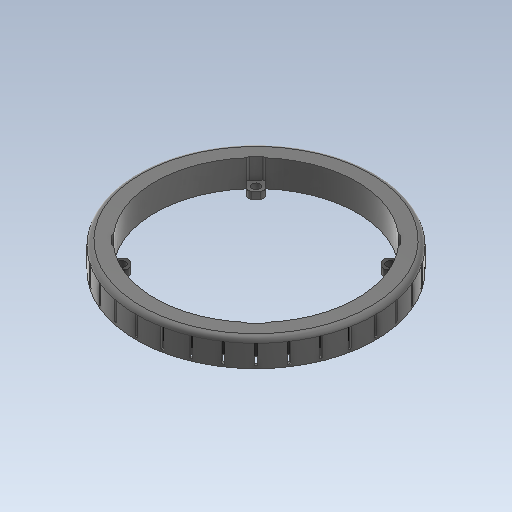
# Autodesk Inventor part: tsop_head
Saved by Autodesk Inventor 2020 (Build 240168000, 168)
## iProperties
Created: 2024-03-11
Part Number: tsop_head
Material: Типовые
Document SubType Name: Modeling
Designer: 4s
Density: 1 g/cm^3
Appearance: Гладкая — черная
Author: 4s
Autodesk Inventor part; units mm, degrees
ref_plane "YZ Plane" through (0, 0, 0) normal (1, 0, 0) x (0, 1, 0)
ref_plane "XZ Plane" through (0, 0, 0) normal (0, 1, 0) x (-1, 0, 0)
ref_plane "XY Plane" through (0, 0, 0) normal (0, 0, 1) x (1, 0, 0)
sketch "Эскиз1" plane through (0, 0, 0) normal (0, 1, 0) x (-1, 0, 0)
  circle A0 centre (0, 0) radius 44 construction
  line L0 (45.8, 2.65) -> (42.7, 2.65)
  line L1 (42.7, 2.65) -> (42.7, -2.65)
  line L2 (42.7, -2.65) -> (45.8, -2.65)
  line L3 (47.8, -0.65) -> (47.8, 0.65)
  line L4 (0, 0) -> (44, 0) construction
  line L5 (0, 0) -> (0, -44) construction
  circle A1 centre (0, 0) radius 49 construction
  circle A2 centre (0, 0) radius 42 construction
  circle A3 centre (0, 0) radius 39 construction
  arc A4 (47.8, 0.65) -> (45.8, 2.65) centre (45.8, 0.65) ccw
  arc A5 (45.8, -2.65) -> (47.8, -0.65) centre (45.8, -0.65) ccw
  line L6 (0, 0) -> (47.8, -0.4878) construction
  line L7 (0, 0) -> (47.8, 0.4878) construction
  line L8 (47.8, 0.4878) -> (48.9974, 0.5)
  line L9 (47.8, -0.4878) -> (48.9974, -0.5)
  line L10 (48.9974, 0.5) -> (49.2908, 0.1398)
  line L11 (49.2908, 0.1398) -> (48.9974, -0.5)
  arc A6 (48.9974, -0.5) -> (48.9974, 0.5) centre (0, 0) ccw
  point P0 (47.8, 2.65)
  point P1 (47.8, -2.65)
  point P2 (49, 0)
  dimension "d0" = 88
  dimension "d1" = 5.3
  dimension "d2" = 1.3
  dimension "d3" = 5.1
  dimension "d4" = 98
  dimension "d5" = 84
  dimension "d6" = 78
  dimension "d16" = 2
  dimension "d17" = 1
  constraints: 24 end point, 11 point on circle, 7 centre point, 6 point on line, 5 coincident, 4 tangent, 2 collinear, 2 horizontal, 2 parallel, 2 perpendicular, 1 equal radius, 1 symmetric about line, 1 other
  measures "d0" diameter of A0
  measures "d1" distance of point (47.8, -2.65) point (47.8, 2.65)
  measures "d2" distance from line of L4.end L1
  measures "d3" distance of L1.end point (47.8, -2.65)
  measures "d4" diameter of A1
  measures "d5" diameter of A2
  measures "d6" diameter of A3
  measures "d16" radius of A4
  measures "d17" distance of L8.end L9.end
sketch "Эскиз2" plane through (0, 0, 0) normal (0, 1, 0) x (-1, 0, 0)
  circle A0 centre (0, 0) radius 49
  circle A1 centre (0, 0) radius 42
  dimension "d7" = 98
  dimension "d8" = 84
  constraints: 2 centre point, 2 coincident
  measures "d7" diameter of A0
  measures "d8" diameter of A1
extrude "Выдавливание1" add sketch "Эскиз2" along normal blind 10
extrude "Выдавливание2" cut sketch "Эскиз1" along normal blind 10 contours A4 L3 A5 L2 L1 L0 | L10 L11 A6
pattern_circular "Круговой массив1" count 32 over 360 about axis through (0, 0, 0) along (0, 1, 0) of "Выдавливание2"
sketch "Эскиз3" plane through (0, 10, 0) normal (0, 1, 0) x (1, 0, 0)
  line L0 (-47.8, -0.65) -> (-47.8, 0.65) construction
  arc A0 (-45.8, 2.65) -> (-47.8, 0.65) centre (-45.8, 0.65) ccw construction
  line L1 (-45.8, 2.65) -> (-42.7, 2.65) construction
  line L2 (-42.7, 2.65) -> (-42.7, -2.65) construction
  line L3 (-42.7, -2.65) -> (-45.8, -2.65) construction
  arc A1 (-47.8, -0.65) -> (-45.8, -2.65) centre (-45.8, -0.65) ccw construction
  line L4 (-46.7547, -9.9628) -> (-47.0083, -8.6878) construction
  arc A2 (-45.437, -6.3361) -> (-47.0083, -8.6878) centre (-45.0468, -8.2976) ccw construction
  line L5 (-45.437, -6.3361) -> (-42.3965, -5.7313) construction
  line L6 (-42.3965, -5.7313) -> (-41.3625, -10.9294) construction
  line L7 (-41.3625, -10.9294) -> (-44.403, -11.5342) construction
  arc A3 (-46.7547, -9.9628) -> (-44.403, -11.5342) centre (-44.7932, -9.5726) ccw construction
  line L8 (-43.9127, -18.8928) -> (-44.4102, -17.6917) construction
  arc A4 (-43.3278, -15.0786) -> (-44.4102, -17.6917) centre (-42.5624, -16.9264) ccw construction
  line L9 (-43.3278, -15.0786) -> (-40.4638, -13.8923) construction
  line L10 (-40.4638, -13.8923) -> (-38.4355, -18.7889) construction
  line L11 (-38.4355, -18.7889) -> (-41.2996, -19.9752) construction
  arc A5 (-43.9127, -18.8928) -> (-41.2996, -19.9752) centre (-42.0649, -18.1274) ccw construction
  line L12 (-39.3831, -27.0967) -> (-40.1054, -26.0158) construction
  arc A6 (-39.5536, -23.2417) -> (-40.1054, -26.0158) centre (-38.4424, -24.9047) ccw construction
  line L13 (-39.5536, -23.2417) -> (-36.976, -21.5195) construction
  line L14 (-36.976, -21.5195) -> (-34.0315, -25.9262) construction
  line L15 (-34.0315, -25.9262) -> (-36.609, -27.6485) construction
  arc A7 (-39.3831, -27.0967) -> (-36.609, -27.6485) centre (-37.7202, -25.9856) ccw construction
  line L16 (-33.3401, -34.2593) -> (-34.2593, -33.3401) construction
  arc A8 (-34.2593, -30.5117) -> (-34.2593, -33.3401) centre (-32.8451, -31.9259) ccw construction
  line L17 (-34.2593, -30.5117) -> (-32.0673, -28.3196) construction
  line L18 (-32.0673, -28.3196) -> (-28.3196, -32.0673) construction
  line L19 (-28.3196, -32.0673) -> (-30.5117, -34.2593) construction
  arc A9 (-33.3401, -34.2593) -> (-30.5117, -34.2593) centre (-31.9259, -32.8451) ccw construction
  line L20 (-26.0158, -40.1054) -> (-27.0967, -39.3831) construction
  arc A10 (-27.6485, -36.609) -> (-27.0967, -39.3831) centre (-25.9856, -37.7202) ccw construction
  line L21 (-27.6485, -36.609) -> (-25.9262, -34.0315) construction
  line L22 (-25.9262, -34.0315) -> (-21.5195, -36.976) construction
  line L23 (-21.5195, -36.976) -> (-23.2417, -39.5536) construction
  arc A11 (-26.0158, -40.1054) -> (-23.2417, -39.5536) centre (-24.9047, -38.4424) ccw construction
  line L24 (-17.6917, -44.4102) -> (-18.8928, -43.9127) construction
  arc A12 (-19.9752, -41.2996) -> (-18.8928, -43.9127) centre (-18.1274, -42.0649) ccw construction
  line L25 (-19.9752, -41.2996) -> (-18.7889, -38.4355) construction
  line L26 (-18.7889, -38.4355) -> (-13.8923, -40.4638) construction
  line L27 (-13.8923, -40.4638) -> (-15.0786, -43.3278) construction
  arc A13 (-17.6917, -44.4102) -> (-15.0786, -43.3278) centre (-16.9264, -42.5624) ccw construction
  line L28 (-8.6878, -47.0083) -> (-9.9628, -46.7547) construction
  arc A14 (-11.5342, -44.403) -> (-9.9628, -46.7547) centre (-9.5726, -44.7932) ccw construction
  line L29 (-11.5342, -44.403) -> (-10.9294, -41.3625) construction
  line L30 (-10.9294, -41.3625) -> (-5.7313, -42.3965) construction
  line L31 (-5.7313, -42.3965) -> (-6.3361, -45.437) construction
  arc A15 (-8.6878, -47.0083) -> (-6.3361, -45.437) centre (-8.2976, -45.0468) ccw construction
  line L32 (0.65, -47.8) -> (-0.65, -47.8) construction
  arc A16 (-2.65, -45.8) -> (-0.65, -47.8) centre (-0.65, -45.8) ccw construction
  line L33 (-2.65, -45.8) -> (-2.65, -42.7) construction
  line L34 (-2.65, -42.7) -> (2.65, -42.7) construction
  line L35 (2.65, -42.7) -> (2.65, -45.8) construction
  arc A17 (0.65, -47.8) -> (2.65, -45.8) centre (0.65, -45.8) ccw construction
  line L36 (9.9628, -46.7547) -> (8.6878, -47.0083) construction
  arc A18 (6.3361, -45.437) -> (8.6878, -47.0083) centre (8.2976, -45.0468) ccw construction
  line L37 (6.3361, -45.437) -> (5.7313, -42.3965) construction
  line L38 (5.7313, -42.3965) -> (10.9294, -41.3625) construction
  line L39 (10.9294, -41.3625) -> (11.5342, -44.403) construction
  arc A19 (9.9628, -46.7547) -> (11.5342, -44.403) centre (9.5726, -44.7932) ccw construction
  line L40 (18.8928, -43.9127) -> (17.6917, -44.4102) construction
  arc A20 (15.0786, -43.3278) -> (17.6917, -44.4102) centre (16.9264, -42.5624) ccw construction
  line L41 (15.0786, -43.3278) -> (13.8923, -40.4638) construction
  line L42 (13.8923, -40.4638) -> (18.7889, -38.4355) construction
  line L43 (18.7889, -38.4355) -> (19.9752, -41.2996) construction
  arc A21 (18.8928, -43.9127) -> (19.9752, -41.2996) centre (18.1274, -42.0649) ccw construction
  line L44 (27.0967, -39.3831) -> (26.0158, -40.1054) construction
  arc A22 (23.2417, -39.5536) -> (26.0158, -40.1054) centre (24.9047, -38.4424) ccw construction
  line L45 (23.2417, -39.5536) -> (21.5195, -36.976) construction
  line L46 (21.5195, -36.976) -> (25.9262, -34.0315) construction
  line L47 (25.9262, -34.0315) -> (27.6485, -36.609) construction
  arc A23 (27.0967, -39.3831) -> (27.6485, -36.609) centre (25.9856, -37.7202) ccw construction
  line L48 (34.2593, -33.3401) -> (33.3401, -34.2593) construction
  arc A24 (30.5117, -34.2593) -> (33.3401, -34.2593) centre (31.9259, -32.8451) ccw construction
  line L49 (30.5117, -34.2593) -> (28.3196, -32.0673) construction
  line L50 (28.3196, -32.0673) -> (32.0673, -28.3196) construction
  line L51 (32.0673, -28.3196) -> (34.2593, -30.5117) construction
  arc A25 (34.2593, -33.3401) -> (34.2593, -30.5117) centre (32.8451, -31.9259) ccw construction
  line L52 (40.1054, -26.0158) -> (39.3831, -27.0967) construction
  arc A26 (36.609, -27.6485) -> (39.3831, -27.0967) centre (37.7202, -25.9856) ccw construction
  line L53 (36.609, -27.6485) -> (34.0315, -25.9262) construction
  line L54 (34.0315, -25.9262) -> (36.976, -21.5195) construction
  line L55 (36.976, -21.5195) -> (39.5536, -23.2417) construction
  arc A27 (40.1054, -26.0158) -> (39.5536, -23.2417) centre (38.4424, -24.9047) ccw construction
  line L56 (44.4102, -17.6917) -> (43.9127, -18.8928) construction
  arc A28 (41.2996, -19.9752) -> (43.9127, -18.8928) centre (42.0649, -18.1274) ccw construction
  line L57 (41.2996, -19.9752) -> (38.4355, -18.7889) construction
  line L58 (38.4355, -18.7889) -> (40.4638, -13.8923) construction
  line L59 (40.4638, -13.8923) -> (43.3278, -15.0786) construction
  arc A29 (44.4102, -17.6917) -> (43.3278, -15.0786) centre (42.5624, -16.9264) ccw construction
  line L60 (47.0083, -8.6878) -> (46.7547, -9.9628) construction
  arc A30 (44.403, -11.5342) -> (46.7547, -9.9628) centre (44.7932, -9.5726) ccw construction
  line L61 (44.403, -11.5342) -> (41.3625, -10.9294) construction
  line L62 (41.3625, -10.9294) -> (42.3965, -5.7313) construction
  line L63 (42.3965, -5.7313) -> (45.437, -6.3361) construction
  arc A31 (47.0083, -8.6878) -> (45.437, -6.3361) centre (45.0468, -8.2976) ccw construction
  line L64 (47.8, 0.65) -> (47.8, -0.65) construction
  arc A32 (45.8, -2.65) -> (47.8, -0.65) centre (45.8, -0.65) ccw construction
  line L65 (45.8, -2.65) -> (42.7, -2.65) construction
  line L66 (42.7, -2.65) -> (42.7, 2.65) construction
  line L67 (42.7, 2.65) -> (45.8, 2.65) construction
  arc A33 (47.8, 0.65) -> (45.8, 2.65) centre (45.8, 0.65) ccw construction
  line L68 (46.7547, 9.9628) -> (47.0083, 8.6878) construction
  arc A34 (45.437, 6.3361) -> (47.0083, 8.6878) centre (45.0468, 8.2976) ccw construction
  line L69 (45.437, 6.3361) -> (42.3965, 5.7313) construction
  line L70 (42.3965, 5.7313) -> (41.3625, 10.9294) construction
  line L71 (41.3625, 10.9294) -> (44.403, 11.5342) construction
  arc A35 (46.7547, 9.9628) -> (44.403, 11.5342) centre (44.7932, 9.5726) ccw construction
  line L72 (43.9127, 18.8928) -> (44.4102, 17.6917) construction
  arc A36 (43.3278, 15.0786) -> (44.4102, 17.6917) centre (42.5624, 16.9264) ccw construction
  line L73 (43.3278, 15.0786) -> (40.4638, 13.8923) construction
  line L74 (40.4638, 13.8923) -> (38.4355, 18.7889) construction
  line L75 (38.4355, 18.7889) -> (41.2996, 19.9752) construction
  arc A37 (43.9127, 18.8928) -> (41.2996, 19.9752) centre (42.0649, 18.1274) ccw construction
  line L76 (39.3831, 27.0967) -> (40.1054, 26.0158) construction
  arc A38 (39.5536, 23.2417) -> (40.1054, 26.0158) centre (38.4424, 24.9047) ccw construction
  line L77 (39.5536, 23.2417) -> (36.976, 21.5195) construction
  line L78 (36.976, 21.5195) -> (34.0315, 25.9262) construction
  line L79 (34.0315, 25.9262) -> (36.609, 27.6485) construction
  arc A39 (39.3831, 27.0967) -> (36.609, 27.6485) centre (37.7202, 25.9856) ccw construction
  line L80 (33.3401, 34.2593) -> (34.2593, 33.3401) construction
  arc A40 (34.2593, 30.5117) -> (34.2593, 33.3401) centre (32.8451, 31.9259) ccw construction
  line L81 (34.2593, 30.5117) -> (32.0673, 28.3196) construction
  line L82 (32.0673, 28.3196) -> (28.3196, 32.0673) construction
  line L83 (28.3196, 32.0673) -> (30.5117, 34.2593) construction
  arc A41 (33.3401, 34.2593) -> (30.5117, 34.2593) centre (31.9259, 32.8451) ccw construction
  line L84 (26.0158, 40.1054) -> (27.0967, 39.3831) construction
  arc A42 (27.6485, 36.609) -> (27.0967, 39.3831) centre (25.9856, 37.7202) ccw construction
  line L85 (27.6485, 36.609) -> (25.9262, 34.0315) construction
  line L86 (25.9262, 34.0315) -> (21.5195, 36.976) construction
  line L87 (21.5195, 36.976) -> (23.2417, 39.5536) construction
  arc A43 (26.0158, 40.1054) -> (23.2417, 39.5536) centre (24.9047, 38.4424) ccw construction
  line L88 (17.6917, 44.4102) -> (18.8928, 43.9127) construction
  arc A44 (19.9752, 41.2996) -> (18.8928, 43.9127) centre (18.1274, 42.0649) ccw construction
  line L89 (19.9752, 41.2996) -> (18.7889, 38.4355) construction
  line L90 (18.7889, 38.4355) -> (13.8923, 40.4638) construction
  line L91 (13.8923, 40.4638) -> (15.0786, 43.3278) construction
  arc A45 (17.6917, 44.4102) -> (15.0786, 43.3278) centre (16.9264, 42.5624) ccw construction
  line L92 (8.6878, 47.0083) -> (9.9628, 46.7547) construction
  arc A46 (11.5342, 44.403) -> (9.9628, 46.7547) centre (9.5726, 44.7932) ccw construction
  line L93 (11.5342, 44.403) -> (10.9294, 41.3625) construction
  line L94 (10.9294, 41.3625) -> (5.7313, 42.3965) construction
  line L95 (5.7313, 42.3965) -> (6.3361, 45.437) construction
  arc A47 (8.6878, 47.0083) -> (6.3361, 45.437) centre (8.2976, 45.0468) ccw construction
  line L96 (-0.65, 47.8) -> (0.65, 47.8) construction
  arc A48 (2.65, 45.8) -> (0.65, 47.8) centre (0.65, 45.8) ccw construction
  line L97 (2.65, 45.8) -> (2.65, 42.7) construction
  line L98 (2.65, 42.7) -> (-2.65, 42.7) construction
  line L99 (-2.65, 42.7) -> (-2.65, 45.8) construction
  arc A49 (-0.65, 47.8) -> (-2.65, 45.8) centre (-0.65, 45.8) ccw construction
  line L100 (-9.9628, 46.7547) -> (-8.6878, 47.0083) construction
  arc A50 (-6.3361, 45.437) -> (-8.6878, 47.0083) centre (-8.2976, 45.0468) ccw construction
  line L101 (-6.3361, 45.437) -> (-5.7313, 42.3965) construction
  line L102 (-5.7313, 42.3965) -> (-10.9294, 41.3625) construction
  line L103 (-10.9294, 41.3625) -> (-11.5342, 44.403) construction
  arc A51 (-9.9628, 46.7547) -> (-11.5342, 44.403) centre (-9.5726, 44.7932) ccw construction
  line L104 (-18.8928, 43.9127) -> (-17.6917, 44.4102) construction
  arc A52 (-15.0786, 43.3278) -> (-17.6917, 44.4102) centre (-16.9264, 42.5624) ccw construction
  line L105 (-15.0786, 43.3278) -> (-13.8923, 40.4638) construction
  line L106 (-13.8923, 40.4638) -> (-18.7889, 38.4355) construction
  line L107 (-18.7889, 38.4355) -> (-19.9752, 41.2996) construction
  arc A53 (-18.8928, 43.9127) -> (-19.9752, 41.2996) centre (-18.1274, 42.0649) ccw construction
  line L108 (-27.0967, 39.3831) -> (-26.0158, 40.1054) construction
  arc A54 (-23.2417, 39.5536) -> (-26.0158, 40.1054) centre (-24.9047, 38.4424) ccw construction
  line L109 (-23.2417, 39.5536) -> (-21.5195, 36.976) construction
  line L110 (-21.5195, 36.976) -> (-25.9262, 34.0315) construction
  line L111 (-25.9262, 34.0315) -> (-27.6485, 36.609) construction
  arc A55 (-27.0967, 39.3831) -> (-27.6485, 36.609) centre (-25.9856, 37.7202) ccw construction
  line L112 (-34.2593, 33.3401) -> (-33.3401, 34.2593) construction
  arc A56 (-30.5117, 34.2593) -> (-33.3401, 34.2593) centre (-31.9259, 32.8451) ccw construction
  line L113 (-30.5117, 34.2593) -> (-28.3196, 32.0673) construction
  line L114 (-28.3196, 32.0673) -> (-32.0673, 28.3196) construction
  line L115 (-32.0673, 28.3196) -> (-34.2593, 30.5117) construction
  arc A57 (-34.2593, 33.3401) -> (-34.2593, 30.5117) centre (-32.8451, 31.9259) ccw construction
  line L116 (-40.1054, 26.0158) -> (-39.3831, 27.0967) construction
  arc A58 (-36.609, 27.6485) -> (-39.3831, 27.0967) centre (-37.7202, 25.9856) ccw construction
  line L117 (-36.609, 27.6485) -> (-34.0315, 25.9262) construction
  line L118 (-34.0315, 25.9262) -> (-36.976, 21.5195) construction
  line L119 (-36.976, 21.5195) -> (-39.5536, 23.2417) construction
  arc A59 (-40.1054, 26.0158) -> (-39.5536, 23.2417) centre (-38.4424, 24.9047) ccw construction
  line L120 (-44.4102, 17.6917) -> (-43.9127, 18.8928) construction
  arc A60 (-41.2996, 19.9752) -> (-43.9127, 18.8928) centre (-42.0649, 18.1274) ccw construction
  line L121 (-41.2996, 19.9752) -> (-38.4355, 18.7889) construction
  line L122 (-38.4355, 18.7889) -> (-40.4638, 13.8923) construction
  line L123 (-40.4638, 13.8923) -> (-43.3278, 15.0786) construction
  arc A61 (-44.4102, 17.6917) -> (-43.3278, 15.0786) centre (-42.5624, 16.9264) ccw construction
  line L124 (-47.0083, 8.6878) -> (-46.7547, 9.9628) construction
  arc A62 (-44.403, 11.5342) -> (-46.7547, 9.9628) centre (-44.7932, 9.5726) ccw construction
  line L125 (-44.403, 11.5342) -> (-41.3625, 10.9294) construction
  line L126 (-41.3625, 10.9294) -> (-42.3965, 5.7313) construction
  line L127 (-42.3965, 5.7313) -> (-45.437, 6.3361) construction
  arc A63 (-47.0083, 8.6878) -> (-45.437, 6.3361) centre (-45.0468, 8.2976) ccw construction
  circle A64 centre (0, 0) radius 42 projected
  circle A65 centre (0, 0) radius 49
  constraints: 1 centre point, 1 coincident
extrude "Выдавливание3" add sketch "Эскиз3" along normal blind 1
fillet "Сопряжение1" radius 2 1 edges at (-49, 11, 0)
extrude "Выдавливание4" cut sketch "Эскиз1" along normal blind 9 contours L8 A6 L9 L3
pattern_circular "Круговой массив2" count 32 over 360 about axis through (0, 0, 0) along (0, 1, 0) of "Выдавливание4"
fillet "Сопряжение2" radius 0.5 1 edges at (-46.8815, 9, -9.3253)
sketch "Эскиз4" plane through (0, 0, 0) normal (0, -1, 0) x (1, 0, 0)
  circle A0 centre (0, 0) radius 39 construction
  line L0 (0, 0) -> (-27.5772, -27.5772) construction
  line L1 (0, 0) -> (39, 0) construction
  circle A1 centre (-27.5772, -27.5772) radius 1.7
  line L2 (0, 0) -> (0, -39) construction
  circle A2 centre (27.5772, -27.5772) radius 1.7
  circle A3 centre (-27.5772, 27.5772) radius 1.7
  circle A4 centre (27.5772, 27.5772) radius 1.7
  line L3 (-31.5793, -27.6902) -> (-28.8146, -24.9255)
  line L4 (-27.6902, -31.5793) -> (-24.9255, -28.8146)
  circle A5 centre (0, 0) radius 42 construction
  circle A6 centre (0, 0) radius 47 construction
  circle A7 centre (0, 0) radius 42 construction
  line L5 (-26.6933, -24.9255) -> (-24.9255, -26.6933)
  arc A8 (-24.9255, -28.8146) -> (-24.9255, -26.6933) centre (-25.9862, -27.7539) ccw
  arc A9 (-26.6933, -24.9255) -> (-28.8146, -24.9255) centre (-27.7539, -25.9862) ccw
  arc A10 (-31.5793, -27.6902) -> (-27.6902, -31.5793) centre (0, 0) ccw
  point P0 (-39, 0)
  point P1 (0, 39)
  point P2 (-27.7539, -23.8649)
  point P3 (-23.8649, -27.7539)
  dimension "d27" = 78
  dimension "d28" = 135
  dimension "d29" = 3.4
  dimension "d30" = 5.5
  dimension "d31" = 2.5
  dimension "d32" = 1.5
  dimension "d33" = 42
  constraints: 12 end point, 11 point on circle, 8 centre point, 5 symmetric about line, 4 point on line, 4 tangent, 2 coincident, 1 equal length, 1 equal radius, 1 horizontal, 1 parallel, 1 vertical, 5 other
  measures "d27" diameter of A0
  measures "d28" angle of L0 L1
  measures "d29" diameter of A1
  measures "d30" distance between parallel lines of L3 L4
  measures "d31" distance from line of L0.end L5
  measures "d32" radius of A8
  measures "d33" radius of A10
extrude "Выдавливание5" add sketch "Эскиз4" along normal blind 0.3 and the other way blind 2.5 contours L3 A9 L5 A8 L4 A10
pattern_circular "Круговой массив3" count 4 over 360 about axis through (0, 0, 0) along (0, 1, 0) of "Выдавливание5"
sketch "Эскиз5" plane through (0, 0, 0) normal (0, -1, 0) x (1, 0, 0)
  circle A0 centre (0, 0) radius 47 construction
  line L0 (-46.7864, -9.8037) -> (-47.9584, -10.0493) construction
  arc A1 (-47.9584, -10.0493) -> (-45.4591, -18.2886) centre (0, 0) ccw construction
  line L1 (-45.4591, -18.2886) -> (-44.3481, -17.8416) construction
  line L2 (-44.3481, -17.8416) -> (-44.4102, -17.6917) construction
  arc A2 (-43.3278, -15.0786) -> (-44.4102, -17.6917) centre (-42.5624, -16.9264) ccw construction
  line L3 (-43.3278, -15.0786) -> (-40.4638, -13.8923) construction
  line L4 (-40.4638, -13.8923) -> (-38.4355, -18.7889) construction
  line L5 (-38.4355, -18.7889) -> (-41.2996, -19.9752) construction
  arc A3 (-43.9127, -18.8928) -> (-41.2996, -19.9752) centre (-42.0649, -18.1274) ccw construction
  line L6 (-43.9127, -18.8928) -> (-43.9748, -18.7429) construction
  line L7 (-43.9748, -18.7429) -> (-45.0764, -19.2125) construction
  arc A4 (-45.0764, -19.2125) -> (-41.0177, -26.8058) centre (0, 0) ccw construction
  line L8 (-41.0177, -26.8058) -> (-40.0152, -26.1507) construction
  line L9 (-40.0152, -26.1507) -> (-40.1054, -26.0158) construction
  arc A5 (-39.5536, -23.2417) -> (-40.1054, -26.0158) centre (-38.4424, -24.9047) ccw construction
  line L10 (-39.5536, -23.2417) -> (-36.976, -21.5195) construction
  line L11 (-36.976, -21.5195) -> (-34.0315, -25.9262) construction
  line L12 (-34.0315, -25.9262) -> (-36.609, -27.6485) construction
  arc A6 (-39.3831, -27.0967) -> (-36.609, -27.6485) centre (-37.7202, -25.9856) ccw construction
  line L13 (-39.3831, -27.0967) -> (-39.4733, -26.9618) construction
  line L14 (-39.4733, -26.9618) -> (-40.4621, -27.6373) construction
  arc A7 (-40.4621, -27.6373) -> (-35, -34.2929) centre (0, 0) ccw construction
  line L15 (-35, -34.2929) -> (-34.1446, -33.4548) construction
  line L16 (-34.1446, -33.4548) -> (-34.2593, -33.3401) construction
  arc A8 (-34.2593, -30.5117) -> (-34.2593, -33.3401) centre (-32.8451, -31.9259) ccw construction
  line L17 (-34.2593, -30.5117) -> (-32.0673, -28.3196) construction
  line L18 (-32.0673, -28.3196) -> (-28.3196, -32.0673) construction
  line L19 (-28.3196, -32.0673) -> (-30.5117, -34.2593) construction
  arc A9 (-33.3401, -34.2593) -> (-30.5117, -34.2593) centre (-31.9259, -32.8451) ccw construction
  line L20 (-33.3401, -34.2593) -> (-33.4548, -34.1446) construction
  line L21 (-33.4548, -34.1446) -> (-34.2929, -35) construction
  arc A10 (-34.2929, -35) -> (-27.6373, -40.4621) centre (0, 0) ccw construction
  line L22 (-27.6373, -40.4621) -> (-26.9618, -39.4733) construction
  line L23 (-26.9618, -39.4733) -> (-27.0967, -39.3831) construction
  arc A11 (-27.6485, -36.609) -> (-27.0967, -39.3831) centre (-25.9856, -37.7202) ccw construction
  line L24 (-27.6485, -36.609) -> (-25.9262, -34.0315) construction
  line L25 (-25.9262, -34.0315) -> (-21.5195, -36.976) construction
  line L26 (-21.5195, -36.976) -> (-23.2417, -39.5536) construction
  arc A12 (-26.0158, -40.1054) -> (-23.2417, -39.5536) centre (-24.9047, -38.4424) ccw construction
  line L27 (-26.0158, -40.1054) -> (-26.1507, -40.0152) construction
  line L28 (-26.1507, -40.0152) -> (-26.8058, -41.0177) construction
  arc A13 (-26.8058, -41.0177) -> (-19.2125, -45.0764) centre (0, 0) ccw construction
  line L29 (-19.2125, -45.0764) -> (-18.7429, -43.9748) construction
  line L30 (-18.7429, -43.9748) -> (-18.8928, -43.9127) construction
  arc A14 (-19.9752, -41.2996) -> (-18.8928, -43.9127) centre (-18.1274, -42.0649) ccw construction
  line L31 (-19.9752, -41.2996) -> (-18.7889, -38.4355) construction
  line L32 (-18.7889, -38.4355) -> (-13.8923, -40.4638) construction
  line L33 (-13.8923, -40.4638) -> (-15.0786, -43.3278) construction
  arc A15 (-17.6917, -44.4102) -> (-15.0786, -43.3278) centre (-16.9264, -42.5624) ccw construction
  line L34 (-17.6917, -44.4102) -> (-17.8416, -44.3481) construction
  line L35 (-17.8416, -44.3481) -> (-18.2886, -45.4591) construction
  arc A16 (-18.2886, -45.4591) -> (-10.0493, -47.9584) centre (0, 0) ccw construction
  line L36 (-10.0493, -47.9584) -> (-9.8037, -46.7864) construction
  line L37 (-9.8037, -46.7864) -> (-9.9628, -46.7547) construction
  arc A17 (-11.5342, -44.403) -> (-9.9628, -46.7547) centre (-9.5726, -44.7932) ccw construction
  line L38 (-11.5342, -44.403) -> (-10.9294, -41.3625) construction
  line L39 (-10.9294, -41.3625) -> (-5.7313, -42.3965) construction
  line L40 (-5.7313, -42.3965) -> (-6.3361, -45.437) construction
  arc A18 (-8.6878, -47.0083) -> (-6.3361, -45.437) centre (-8.2976, -45.0468) ccw construction
  line L41 (-8.6878, -47.0083) -> (-8.8469, -46.9767) construction
  line L42 (-8.8469, -46.9767) -> (-9.0685, -48.1535) construction
  arc A19 (-9.0685, -48.1535) -> (-0.5, -48.9974) centre (0, 0) ccw construction
  line L43 (-0.5, -48.9974) -> (-0.4878, -47.8) construction
  line L44 (-0.4878, -47.8) -> (-0.65, -47.8) construction
  arc A20 (-2.65, -45.8) -> (-0.65, -47.8) centre (-0.65, -45.8) ccw construction
  line L45 (-2.65, -45.8) -> (-2.65, -42.7) construction
  line L46 (-2.65, -42.7) -> (2.65, -42.7) construction
  line L47 (2.65, -42.7) -> (2.65, -45.8) construction
  arc A21 (0.65, -47.8) -> (2.65, -45.8) centre (0.65, -45.8) ccw construction
  line L48 (0.65, -47.8) -> (0.4878, -47.8) construction
  line L49 (0.4878, -47.8) -> (0.5, -48.9974) construction
  arc A22 (0.5, -48.9974) -> (9.0685, -48.1535) centre (0, 0) ccw construction
  line L50 (9.0685, -48.1535) -> (8.8469, -46.9767) construction
  line L51 (8.8469, -46.9767) -> (8.6878, -47.0083) construction
  arc A23 (6.3361, -45.437) -> (8.6878, -47.0083) centre (8.2976, -45.0468) ccw construction
  line L52 (6.3361, -45.437) -> (5.7313, -42.3965) construction
  line L53 (5.7313, -42.3965) -> (10.9294, -41.3625) construction
  line L54 (10.9294, -41.3625) -> (11.5342, -44.403) construction
  arc A24 (9.9628, -46.7547) -> (11.5342, -44.403) centre (9.5726, -44.7932) ccw construction
  line L55 (9.9628, -46.7547) -> (9.8037, -46.7864) construction
  line L56 (9.8037, -46.7864) -> (10.0493, -47.9584) construction
  arc A25 (10.0493, -47.9584) -> (18.2886, -45.4591) centre (0, 0) ccw construction
  line L57 (18.2886, -45.4591) -> (17.8416, -44.3481) construction
  line L58 (17.8416, -44.3481) -> (17.6917, -44.4102) construction
  arc A26 (15.0786, -43.3278) -> (17.6917, -44.4102) centre (16.9264, -42.5624) ccw construction
  line L59 (15.0786, -43.3278) -> (13.8923, -40.4638) construction
  line L60 (13.8923, -40.4638) -> (18.7889, -38.4355) construction
  line L61 (18.7889, -38.4355) -> (19.9752, -41.2996) construction
  arc A27 (18.8928, -43.9127) -> (19.9752, -41.2996) centre (18.1274, -42.0649) ccw construction
  line L62 (18.8928, -43.9127) -> (18.7429, -43.9748) construction
  line L63 (18.7429, -43.9748) -> (19.2125, -45.0764) construction
  arc A28 (19.2125, -45.0764) -> (26.8058, -41.0177) centre (0, 0) ccw construction
  line L64 (26.8058, -41.0177) -> (26.1507, -40.0152) construction
  line L65 (26.1507, -40.0152) -> (26.0158, -40.1054) construction
  arc A29 (23.2417, -39.5536) -> (26.0158, -40.1054) centre (24.9047, -38.4424) ccw construction
  line L66 (23.2417, -39.5536) -> (21.5195, -36.976) construction
  line L67 (21.5195, -36.976) -> (25.9262, -34.0315) construction
  line L68 (25.9262, -34.0315) -> (27.6485, -36.609) construction
  arc A30 (27.0967, -39.3831) -> (27.6485, -36.609) centre (25.9856, -37.7202) ccw construction
  line L69 (27.0967, -39.3831) -> (26.9618, -39.4733) construction
  line L70 (26.9618, -39.4733) -> (27.6373, -40.4621) construction
  arc A31 (27.6373, -40.4621) -> (34.2929, -35) centre (0, 0) ccw construction
  line L71 (34.2929, -35) -> (33.4548, -34.1446) construction
  line L72 (33.4548, -34.1446) -> (33.3401, -34.2593) construction
  arc A32 (30.5117, -34.2593) -> (33.3401, -34.2593) centre (31.9259, -32.8451) ccw construction
  line L73 (30.5117, -34.2593) -> (28.3196, -32.0673) construction
  line L74 (28.3196, -32.0673) -> (32.0673, -28.3196) construction
  line L75 (32.0673, -28.3196) -> (34.2593, -30.5117) construction
  arc A33 (34.2593, -33.3401) -> (34.2593, -30.5117) centre (32.8451, -31.9259) ccw construction
  line L76 (34.2593, -33.3401) -> (34.1446, -33.4548) construction
  line L77 (34.1446, -33.4548) -> (35, -34.2929) construction
  arc A34 (35, -34.2929) -> (40.4621, -27.6373) centre (0, 0) ccw construction
  line L78 (40.4621, -27.6373) -> (39.4733, -26.9618) construction
  line L79 (39.4733, -26.9618) -> (39.3831, -27.0967) construction
  arc A35 (36.609, -27.6485) -> (39.3831, -27.0967) centre (37.7202, -25.9856) ccw construction
  line L80 (36.609, -27.6485) -> (34.0315, -25.9262) construction
  line L81 (34.0315, -25.9262) -> (36.976, -21.5195) construction
  line L82 (36.976, -21.5195) -> (39.5536, -23.2417) construction
  arc A36 (40.1054, -26.0158) -> (39.5536, -23.2417) centre (38.4424, -24.9047) ccw construction
  line L83 (40.1054, -26.0158) -> (40.0152, -26.1507) construction
  line L84 (40.0152, -26.1507) -> (41.0177, -26.8058) construction
  arc A37 (41.0177, -26.8058) -> (45.0764, -19.2125) centre (0, 0) ccw construction
  line L85 (45.0764, -19.2125) -> (43.9748, -18.7429) construction
  line L86 (43.9748, -18.7429) -> (43.9127, -18.8928) construction
  arc A38 (41.2996, -19.9752) -> (43.9127, -18.8928) centre (42.0649, -18.1274) ccw construction
  line L87 (41.2996, -19.9752) -> (38.4355, -18.7889) construction
  line L88 (38.4355, -18.7889) -> (40.4638, -13.8923) construction
  line L89 (40.4638, -13.8923) -> (43.3278, -15.0786) construction
  arc A39 (44.4102, -17.6917) -> (43.3278, -15.0786) centre (42.5624, -16.9264) ccw construction
  line L90 (44.4102, -17.6917) -> (44.3481, -17.8416) construction
  line L91 (44.3481, -17.8416) -> (45.4591, -18.2886) construction
  arc A40 (45.4591, -18.2886) -> (47.9584, -10.0493) centre (0, 0) ccw construction
  line L92 (47.9584, -10.0493) -> (46.7864, -9.8037) construction
  line L93 (46.7864, -9.8037) -> (46.7547, -9.9628) construction
  arc A41 (44.403, -11.5342) -> (46.7547, -9.9628) centre (44.7932, -9.5726) ccw construction
  line L94 (44.403, -11.5342) -> (41.3625, -10.9294) construction
  line L95 (41.3625, -10.9294) -> (42.3965, -5.7313) construction
  line L96 (42.3965, -5.7313) -> (45.437, -6.3361) construction
  arc A42 (47.0083, -8.6878) -> (45.437, -6.3361) centre (45.0468, -8.2976) ccw construction
  line L97 (47.0083, -8.6878) -> (46.9767, -8.8469) construction
  line L98 (46.9767, -8.8469) -> (48.1535, -9.0685) construction
  arc A43 (48.1535, -9.0685) -> (48.9974, -0.5) centre (0, 0) ccw construction
  line L99 (48.9974, -0.5) -> (47.8, -0.4878) construction
  line L100 (47.8, -0.4878) -> (47.8, -0.65) construction
  arc A44 (45.8, -2.65) -> (47.8, -0.65) centre (45.8, -0.65) ccw construction
  line L101 (45.8, -2.65) -> (42.7, -2.65) construction
  line L102 (42.7, -2.65) -> (42.7, 2.65) construction
  line L103 (42.7, 2.65) -> (45.8, 2.65) construction
  arc A45 (47.8, 0.65) -> (45.8, 2.65) centre (45.8, 0.65) ccw construction
  line L104 (47.8, 0.65) -> (47.8, 0.4878) construction
  line L105 (47.8, 0.4878) -> (48.9974, 0.5) construction
  arc A46 (48.9974, 0.5) -> (48.1535, 9.0685) centre (0, 0) ccw construction
  line L106 (48.1535, 9.0685) -> (46.9767, 8.8469) construction
  line L107 (46.9767, 8.8469) -> (47.0083, 8.6878) construction
  arc A47 (45.437, 6.3361) -> (47.0083, 8.6878) centre (45.0468, 8.2976) ccw construction
  line L108 (45.437, 6.3361) -> (42.3965, 5.7313) construction
  line L109 (42.3965, 5.7313) -> (41.3625, 10.9294) construction
  line L110 (41.3625, 10.9294) -> (44.403, 11.5342) construction
  arc A48 (46.7547, 9.9628) -> (44.403, 11.5342) centre (44.7932, 9.5726) ccw construction
  line L111 (46.7547, 9.9628) -> (46.7864, 9.8037) construction
  line L112 (46.7864, 9.8037) -> (47.9584, 10.0493) construction
  arc A49 (47.9584, 10.0493) -> (45.4591, 18.2886) centre (0, 0) ccw construction
  line L113 (45.4591, 18.2886) -> (44.3481, 17.8416) construction
  line L114 (44.3481, 17.8416) -> (44.4102, 17.6917) construction
  arc A50 (43.3278, 15.0786) -> (44.4102, 17.6917) centre (42.5624, 16.9264) ccw construction
  line L115 (43.3278, 15.0786) -> (40.4638, 13.8923) construction
  line L116 (40.4638, 13.8923) -> (38.4355, 18.7889) construction
  line L117 (38.4355, 18.7889) -> (41.2996, 19.9752) construction
  arc A51 (43.9127, 18.8928) -> (41.2996, 19.9752) centre (42.0649, 18.1274) ccw construction
  line L118 (43.9127, 18.8928) -> (43.9748, 18.7429) construction
  line L119 (43.9748, 18.7429) -> (45.0764, 19.2125) construction
  arc A52 (45.0764, 19.2125) -> (41.0177, 26.8058) centre (0, 0) ccw construction
  line L120 (41.0177, 26.8058) -> (40.0152, 26.1507) construction
  line L121 (40.0152, 26.1507) -> (40.1054, 26.0158) construction
  arc A53 (39.5536, 23.2417) -> (40.1054, 26.0158) centre (38.4424, 24.9047) ccw construction
  line L122 (39.5536, 23.2417) -> (36.976, 21.5195) construction
  line L123 (36.976, 21.5195) -> (34.0315, 25.9262) construction
  line L124 (34.0315, 25.9262) -> (36.609, 27.6485) construction
  arc A54 (39.3831, 27.0967) -> (36.609, 27.6485) centre (37.7202, 25.9856) ccw construction
  line L125 (39.3831, 27.0967) -> (39.4733, 26.9618) construction
  line L126 (39.4733, 26.9618) -> (40.4621, 27.6373) construction
  arc A55 (40.4621, 27.6373) -> (35, 34.2929) centre (0, 0) ccw construction
  line L127 (35, 34.2929) -> (34.1446, 33.4548) construction
  line L128 (34.1446, 33.4548) -> (34.2593, 33.3401) construction
  arc A56 (34.2593, 30.5117) -> (34.2593, 33.3401) centre (32.8451, 31.9259) ccw construction
  line L129 (34.2593, 30.5117) -> (32.0673, 28.3196) construction
  line L130 (32.0673, 28.3196) -> (28.3196, 32.0673) construction
  line L131 (28.3196, 32.0673) -> (30.5117, 34.2593) construction
  arc A57 (33.3401, 34.2593) -> (30.5117, 34.2593) centre (31.9259, 32.8451) ccw construction
  line L132 (33.3401, 34.2593) -> (33.4548, 34.1446) construction
  line L133 (33.4548, 34.1446) -> (34.2929, 35) construction
  arc A58 (34.2929, 35) -> (27.6373, 40.4621) centre (0, 0) ccw construction
  line L134 (27.6373, 40.4621) -> (26.9618, 39.4733) construction
  line L135 (26.9618, 39.4733) -> (27.0967, 39.3831) construction
  arc A59 (27.6485, 36.609) -> (27.0967, 39.3831) centre (25.9856, 37.7202) ccw construction
  line L136 (27.6485, 36.609) -> (25.9262, 34.0315) construction
  line L137 (25.9262, 34.0315) -> (21.5195, 36.976) construction
  line L138 (21.5195, 36.976) -> (23.2417, 39.5536) construction
  arc A60 (26.0158, 40.1054) -> (23.2417, 39.5536) centre (24.9047, 38.4424) ccw construction
  line L139 (26.0158, 40.1054) -> (26.1507, 40.0152) construction
  line L140 (26.1507, 40.0152) -> (26.8058, 41.0177) construction
  arc A61 (26.8058, 41.0177) -> (19.2125, 45.0764) centre (0, 0) ccw construction
  line L141 (19.2125, 45.0764) -> (18.7429, 43.9748) construction
  line L142 (18.7429, 43.9748) -> (18.8928, 43.9127) construction
  arc A62 (19.9752, 41.2996) -> (18.8928, 43.9127) centre (18.1274, 42.0649) ccw construction
  line L143 (19.9752, 41.2996) -> (18.7889, 38.4355) construction
  line L144 (18.7889, 38.4355) -> (13.8923, 40.4638) construction
  line L145 (13.8923, 40.4638) -> (15.0786, 43.3278) construction
  arc A63 (17.6917, 44.4102) -> (15.0786, 43.3278) centre (16.9264, 42.5624) ccw construction
  line L146 (17.6917, 44.4102) -> (17.8416, 44.3481) construction
  line L147 (17.8416, 44.3481) -> (18.2886, 45.4591) construction
  arc A64 (18.2886, 45.4591) -> (10.0493, 47.9584) centre (0, 0) ccw construction
  line L148 (10.0493, 47.9584) -> (9.8037, 46.7864) construction
  line L149 (9.8037, 46.7864) -> (9.9628, 46.7547) construction
  arc A65 (11.5342, 44.403) -> (9.9628, 46.7547) centre (9.5726, 44.7932) ccw construction
  line L150 (11.5342, 44.403) -> (10.9294, 41.3625) construction
  line L151 (10.9294, 41.3625) -> (5.7313, 42.3965) construction
  line L152 (5.7313, 42.3965) -> (6.3361, 45.437) construction
  arc A66 (8.6878, 47.0083) -> (6.3361, 45.437) centre (8.2976, 45.0468) ccw construction
  line L153 (8.6878, 47.0083) -> (8.8469, 46.9767) construction
  line L154 (8.8469, 46.9767) -> (9.0685, 48.1535) construction
  arc A67 (9.0685, 48.1535) -> (0.5, 48.9974) centre (0, 0) ccw construction
  line L155 (0.5, 48.9974) -> (0.4878, 47.8) construction
  line L156 (0.4878, 47.8) -> (0.65, 47.8) construction
  arc A68 (2.65, 45.8) -> (0.65, 47.8) centre (0.65, 45.8) ccw construction
  line L157 (2.65, 45.8) -> (2.65, 42.7) construction
  line L158 (2.65, 42.7) -> (-2.65, 42.7) construction
  line L159 (-2.65, 42.7) -> (-2.65, 45.8) construction
  arc A69 (-0.65, 47.8) -> (-2.65, 45.8) centre (-0.65, 45.8) ccw construction
  line L160 (-0.65, 47.8) -> (-0.4878, 47.8) construction
  line L161 (-0.4878, 47.8) -> (-0.5, 48.9974) construction
  arc A70 (-0.5, 48.9974) -> (-9.0685, 48.1535) centre (0, 0) ccw construction
  line L162 (-9.0685, 48.1535) -> (-8.8469, 46.9767) construction
  line L163 (-8.8469, 46.9767) -> (-8.6878, 47.0083) construction
  arc A71 (-6.3361, 45.437) -> (-8.6878, 47.0083) centre (-8.2976, 45.0468) ccw construction
  line L164 (-6.3361, 45.437) -> (-5.7313, 42.3965) construction
  line L165 (-5.7313, 42.3965) -> (-10.9294, 41.3625) construction
  line L166 (-10.9294, 41.3625) -> (-11.5342, 44.403) construction
  arc A72 (-9.9628, 46.7547) -> (-11.5342, 44.403) centre (-9.5726, 44.7932) ccw construction
  line L167 (-9.9628, 46.7547) -> (-9.8037, 46.7864) construction
  line L168 (-9.8037, 46.7864) -> (-10.0493, 47.9584) construction
  arc A73 (-10.0493, 47.9584) -> (-18.2886, 45.4591) centre (0, 0) ccw construction
  line L169 (-18.2886, 45.4591) -> (-17.8416, 44.3481) construction
  line L170 (-17.8416, 44.3481) -> (-17.6917, 44.4102) construction
  arc A74 (-15.0786, 43.3278) -> (-17.6917, 44.4102) centre (-16.9264, 42.5624) ccw construction
  line L171 (-15.0786, 43.3278) -> (-13.8923, 40.4638) construction
  line L172 (-13.8923, 40.4638) -> (-18.7889, 38.4355) construction
  line L173 (-18.7889, 38.4355) -> (-19.9752, 41.2996) construction
  arc A75 (-18.8928, 43.9127) -> (-19.9752, 41.2996) centre (-18.1274, 42.0649) ccw construction
  line L174 (-18.8928, 43.9127) -> (-18.7429, 43.9748) construction
  line L175 (-18.7429, 43.9748) -> (-19.2125, 45.0764) construction
  arc A76 (-19.2125, 45.0764) -> (-26.8058, 41.0177) centre (0, 0) ccw construction
  line L176 (-26.8058, 41.0177) -> (-26.1507, 40.0152) construction
  line L177 (-26.1507, 40.0152) -> (-26.0158, 40.1054) construction
  arc A77 (-23.2417, 39.5536) -> (-26.0158, 40.1054) centre (-24.9047, 38.4424) ccw construction
  line L178 (-23.2417, 39.5536) -> (-21.5195, 36.976) construction
  line L179 (-21.5195, 36.976) -> (-25.9262, 34.0315) construction
  line L180 (-25.9262, 34.0315) -> (-27.6485, 36.609) construction
  arc A78 (-27.0967, 39.3831) -> (-27.6485, 36.609) centre (-25.9856, 37.7202) ccw construction
  line L181 (-27.0967, 39.3831) -> (-26.9618, 39.4733) construction
  line L182 (-26.9618, 39.4733) -> (-27.6373, 40.4621) construction
  arc A79 (-27.6373, 40.4621) -> (-34.2929, 35) centre (0, 0) ccw construction
  line L183 (-34.2929, 35) -> (-33.4548, 34.1446) construction
  line L184 (-33.4548, 34.1446) -> (-33.3401, 34.2593) construction
  arc A80 (-30.5117, 34.2593) -> (-33.3401, 34.2593) centre (-31.9259, 32.8451) ccw construction
  line L185 (-30.5117, 34.2593) -> (-28.3196, 32.0673) construction
  line L186 (-28.3196, 32.0673) -> (-32.0673, 28.3196) construction
  line L187 (-32.0673, 28.3196) -> (-34.2593, 30.5117) construction
  arc A81 (-34.2593, 33.3401) -> (-34.2593, 30.5117) centre (-32.8451, 31.9259) ccw construction
  line L188 (-34.2593, 33.3401) -> (-34.1446, 33.4548) construction
  line L189 (-34.1446, 33.4548) -> (-35, 34.2929) construction
  arc A82 (-35, 34.2929) -> (-40.4621, 27.6373) centre (0, 0) ccw construction
  line L190 (-40.4621, 27.6373) -> (-39.4733, 26.9618) construction
  line L191 (-39.4733, 26.9618) -> (-39.3831, 27.0967) construction
  arc A83 (-36.609, 27.6485) -> (-39.3831, 27.0967) centre (-37.7202, 25.9856) ccw construction
  line L192 (-36.609, 27.6485) -> (-34.0315, 25.9262) construction
  line L193 (-34.0315, 25.9262) -> (-36.976, 21.5195) construction
  line L194 (-36.976, 21.5195) -> (-39.5536, 23.2417) construction
  arc A84 (-40.1054, 26.0158) -> (-39.5536, 23.2417) centre (-38.4424, 24.9047) ccw construction
  line L195 (-40.1054, 26.0158) -> (-40.0152, 26.1507) construction
  line L196 (-40.0152, 26.1507) -> (-41.0177, 26.8058) construction
  arc A85 (-41.0177, 26.8058) -> (-45.0764, 19.2125) centre (0, 0) ccw construction
  line L197 (-45.0764, 19.2125) -> (-43.9748, 18.7429) construction
  line L198 (-43.9748, 18.7429) -> (-43.9127, 18.8928) construction
  arc A86 (-41.2996, 19.9752) -> (-43.9127, 18.8928) centre (-42.0649, 18.1274) ccw construction
  line L199 (-41.2996, 19.9752) -> (-38.4355, 18.7889) construction
  line L200 (-38.4355, 18.7889) -> (-40.4638, 13.8923) construction
  line L201 (-40.4638, 13.8923) -> (-43.3278, 15.0786) construction
  arc A87 (-44.4102, 17.6917) -> (-43.3278, 15.0786) centre (-42.5624, 16.9264) ccw construction
  line L202 (-44.4102, 17.6917) -> (-44.3481, 17.8416) construction
  line L203 (-44.3481, 17.8416) -> (-45.4591, 18.2886) construction
  arc A88 (-45.4591, 18.2886) -> (-47.9584, 10.0493) centre (0, 0) ccw construction
  line L204 (-47.9584, 10.0493) -> (-46.7864, 9.8037) construction
  line L205 (-46.7864, 9.8037) -> (-46.7547, 9.9628) construction
  arc A89 (-44.403, 11.5342) -> (-46.7547, 9.9628) centre (-44.7932, 9.5726) ccw construction
  line L206 (-44.403, 11.5342) -> (-41.3625, 10.9294) construction
  line L207 (-41.3625, 10.9294) -> (-42.3965, 5.7313) construction
  line L208 (-42.3965, 5.7313) -> (-45.437, 6.3361) construction
  arc A90 (-47.0083, 8.6878) -> (-45.437, 6.3361) centre (-45.0468, 8.2976) ccw construction
  line L209 (-47.0083, 8.6878) -> (-46.9767, 8.8469) construction
  line L210 (-46.9767, 8.8469) -> (-48.1535, 9.0685) construction
  arc A91 (-48.1535, 9.0685) -> (-48.9974, 0.5) centre (0, 0) ccw construction
  line L211 (-48.9974, 0.5) -> (-47.8, 0.4878) construction
  line L212 (-47.8, 0.4878) -> (-47.8, 0.65) construction
  arc A92 (-45.8, 2.65) -> (-47.8, 0.65) centre (-45.8, 0.65) ccw construction
  line L213 (-45.8, 2.65) -> (-42.7, 2.65) construction
  line L214 (-42.7, 2.65) -> (-42.7, -2.65) construction
  line L215 (-42.7, -2.65) -> (-45.8, -2.65) construction
  arc A93 (-47.8, -0.65) -> (-45.8, -2.65) centre (-45.8, -0.65) ccw construction
  line L216 (-47.8, -0.65) -> (-47.8, -0.4878) construction
  line L217 (-47.8, -0.4878) -> (-48.9974, -0.5) construction
  arc A94 (-48.9974, -0.5) -> (-48.1535, -9.0685) centre (0, 0) ccw construction
  line L218 (-48.1535, -9.0685) -> (-46.9767, -8.8469) construction
  line L219 (-46.9767, -8.8469) -> (-47.0083, -8.6878) construction
  arc A95 (-45.437, -6.3361) -> (-47.0083, -8.6878) centre (-45.0468, -8.2976) ccw construction
  line L220 (-45.437, -6.3361) -> (-42.3965, -5.7313) construction
  line L221 (-42.3965, -5.7313) -> (-41.3625, -10.9294) construction
  line L222 (-41.3625, -10.9294) -> (-44.403, -11.5342) construction
  arc A96 (-46.7547, -9.9628) -> (-44.403, -11.5342) centre (-44.7932, -9.5726) ccw construction
  line L223 (-46.7547, -9.9628) -> (-46.7864, -9.8037) construction
  arc A97 (-27.6902, -31.5793) -> (27.6902, -31.5793) centre (0, 0) ccw projected
  arc A98 (-31.5793, -27.6902) -> (-27.6902, -31.5793) centre (0, 0) ccw construction
  arc A99 (-31.5793, 27.6902) -> (-31.5793, -27.6902) centre (0, 0) ccw projected
  arc A100 (-27.6902, 31.5793) -> (-31.5793, 27.6902) centre (0, 0) ccw construction
  arc A101 (27.6902, 31.5793) -> (-27.6902, 31.5793) centre (0, 0) ccw projected
  arc A102 (31.5793, 27.6902) -> (27.6902, 31.5793) centre (0, 0) ccw construction
  arc A103 (31.5793, -27.6902) -> (31.5793, 27.6902) centre (0, 0) ccw projected
  arc A104 (27.6902, -31.5793) -> (31.5793, -27.6902) centre (0, 0) ccw construction
  line L224 (27.6902, 31.5793) -> (24.9255, 28.8146) projected
  arc A105 (24.9255, 28.8146) -> (24.9255, 26.6933) centre (25.9862, 27.7539) ccw projected
  line L225 (24.9255, 26.6933) -> (26.6933, 24.9255) projected
  arc A106 (26.6933, 24.9255) -> (28.8146, 24.9255) centre (27.7539, 25.9862) ccw projected
  line L226 (28.8146, 24.9255) -> (31.5793, 27.6902) projected
  arc A107 (31.5793, 27.6902) -> (27.6902, 31.5793) centre (0, 0) ccw construction
  circle A108 centre (27.5772, 27.5772) radius 1.7 projected
  line L227 (31.5793, -27.6902) -> (28.8146, -24.9255) projected
  arc A109 (28.8146, -24.9255) -> (26.6933, -24.9255) centre (27.7539, -25.9862) ccw projected
  line L228 (26.6933, -24.9255) -> (24.9255, -26.6933) projected
  arc A110 (24.9255, -26.6933) -> (24.9255, -28.8146) centre (25.9862, -27.7539) ccw projected
  line L229 (24.9255, -28.8146) -> (27.6902, -31.5793) projected
  arc A111 (27.6902, -31.5793) -> (31.5793, -27.6902) centre (0, 0) ccw construction
  circle A112 centre (27.5772, -27.5772) radius 1.7 projected
  line L230 (-27.6902, -31.5793) -> (-24.9255, -28.8146) projected
  arc A113 (-24.9255, -28.8146) -> (-24.9255, -26.6933) centre (-25.9862, -27.7539) ccw projected
  line L231 (-24.9255, -26.6933) -> (-26.6933, -24.9255) projected
  arc A114 (-26.6933, -24.9255) -> (-28.8146, -24.9255) centre (-27.7539, -25.9862) ccw projected
  line L232 (-28.8146, -24.9255) -> (-31.5793, -27.6902) projected
  arc A115 (-31.5793, -27.6902) -> (-27.6902, -31.5793) centre (0, 0) ccw construction
  circle A116 centre (-27.5772, -27.5772) radius 1.7 projected
  line L233 (-31.5793, 27.6902) -> (-28.8146, 24.9255) projected
  arc A117 (-28.8146, 24.9255) -> (-26.6933, 24.9255) centre (-27.7539, 25.9862) ccw projected
  line L234 (-26.6933, 24.9255) -> (-24.9255, 26.6933) projected
  arc A118 (-24.9255, 26.6933) -> (-24.9255, 28.8146) centre (-25.9862, 27.7539) ccw projected
  line L235 (-24.9255, 28.8146) -> (-27.6902, 31.5793) projected
  arc A119 (-27.6902, 31.5793) -> (-31.5793, 27.6902) centre (0, 0) ccw construction
  circle A120 centre (-27.5772, 27.5772) radius 1.7 projected
  arc A121 (-27.265, 31.1541) -> (-31.1541, 27.265) centre (0, 0) ccw construction
  arc A122 (27.265, 31.1541) -> (-27.265, 31.1541) centre (0, 0) ccw
  arc A123 (31.1541, -27.265) -> (31.1541, 27.265) centre (0, 0) ccw
  arc A124 (31.1541, 27.265) -> (27.265, 31.1541) centre (0, 0) ccw construction
  arc A125 (27.265, -31.1541) -> (31.1541, -27.265) centre (0, 0) ccw construction
  arc A126 (-27.265, -31.1541) -> (27.265, -31.1541) centre (0, 0) ccw
  arc A127 (-31.1541, -27.265) -> (-27.265, -31.1541) centre (0, 0) ccw
  arc A128 (-31.1541, 27.265) -> (-31.1541, -27.265) centre (0, 0) ccw
  dimension "d41" = 0.6
  constraints: 16 point on circle, 8 centre point, 8 point on line, 1 coincident
  measures "d41" radial gap between concentric circles of A101 A121
extrude "Выдавливание6" add sketch "Эскиз5" against normal up to surface (11 mm away) contours L230 A126 L229 A97 | L232 A99 L233 A128 | A123 L226 A103 L227 | L235 A101 L224 A122
fillet "Сопряжение3" radius 1 8 edges at (-27.6902, 6.75, -31.5793) (-31.5793, 6.75, -27.6902) (-31.5793, 6.75, 27.6902) (-27.6902, 6.75, 31.5793) (31.5793, 6.75, 27.6902) (27.6902, 6.75, 31.5793) (27.6902, 6.75, -31.5793) (31.5793, 6.75, -27.6902)
sketch "Эскиз6" plane through (-26.9618, 0, 39.4733) normal (0.8257572, 0, 0.5640257) x (0.5640257, 0, -0.8257572)
  point P0 (47.8025, 0)
extrude "Выдавливание7" add sketch "Эскиз1" along normal blind 1 contours L8 A6 L9 L3
pattern_circular "Круговой массив4" count 32 over 360 about axis through (0, 0, 0) along (0, 1, 0) of "Выдавливание7"
